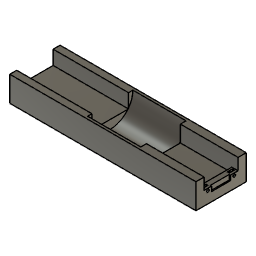
LabelStamp (Autodesk Fusion 360 design; units mm, degrees)
Autodesk Fusion 360 part; units mm, degrees
sketch "スケッチ1" plane through (0, 0, 0) normal (0, 0, 1) x (1, 0, 0)
  line L0 (0, 0) -> (148.1, 0)
  line L1 (148.1, 0) -> (148.1, 40)
  line L2 (148.1, 40) -> (0, 40)
  line L3 (0, 40) -> (0, 0)
  dimension "d1" = 148.1
  dimension "d2" = 40
  constraint horizontal L0
  constraint vertical L1
  constraint horizontal L2
  constraint vertical L3
  constraint coincident L0.start L3.end
  measures "d1" distance of L0.start L0.end
  measures "d2" distance of L0.start L2.end
extrude "押し出し1" add sketch "スケッチ1" along normal blind 8.8
sketch "スケッチ2" plane through (0, 0, 8.8) normal (0, 0, 1) x (-1, 0, 0)
  line L0 (0, -40) -> (0, 0)
  line L1 (0, 0) -> (-148.1, 0)
  line L2 (-148.1, 0) -> (-148.1, -40)
  line L3 (-148.1, -40) -> (0, -40)
  line L4 (-148.1, -40) -> (-102.2, -40)
  line L5 (-102.2, -40) -> (-102.2, -33.5)
  line L6 (-102.2, -33.5) -> (-148.1, -33.5)
  line L7 (-148.1, -33.5) -> (-148.1, -40)
  line L8 (-148.1, 0) -> (-102.2, 0)
  line L9 (-102.2, 0) -> (-102.2, -6.5)
  line L10 (-102.2, -6.5) -> (-148.1, -6.5)
  line L11 (-148.1, -6.5) -> (-148.1, 0)
  line L12 (0, -40) -> (-59.9, -40)
  line L13 (-59.9, -40) -> (-59.9, -34.5)
  line L14 (-59.9, -34.5) -> (0, -34.5)
  line L15 (0, -34.5) -> (0, -40)
  line L16 (0, 0) -> (-59.9, 0)
  line L17 (-59.9, 0) -> (-59.9, -5.5)
  line L18 (-59.9, -5.5) -> (0, -5.5)
  line L19 (0, -5.5) -> (0, 0)
  line L20 (-59.9, -40) -> (-102.2, -40)
  line L21 (-102.2, -40) -> (-102.2, 0)
  line L22 (-102.2, 0) -> (-59.9, 0)
  line L23 (-59.9, 0) -> (-59.9, -40)
  dimension "d5" = 45.9
  dimension "d6" = 6.5
  dimension "d7" = 45.9
  dimension "d8" = 6.5
  dimension "d9" = 59.9
  dimension "d10" = 5.5
  dimension "d11" = 59.9
  dimension "d12" = 5.5
  constraint horizontal L4
  constraint vertical L5
  constraint horizontal L6
  constraint vertical L7
  constraint coincident L2.end L3.start
  constraint horizontal L8
  constraint vertical L9
  constraint horizontal L10
  constraint vertical L11
  constraint coincident L1.end L2.start
  constraint horizontal L12
  constraint vertical L13
  constraint horizontal L14
  constraint vertical L15
  constraint coincident L0.start L3.end
  constraint horizontal L16
  constraint vertical L17
  constraint horizontal L18
  constraint vertical L19
  constraint coincident L0.end L1.start
  constraint horizontal L20
  constraint vertical L21
  constraint horizontal L22
  constraint vertical L23
  measures "d5" distance of L2.end L4.end
  measures "d6" distance of L2.end L6.end
  measures "d7" distance of L1.end L8.end
  measures "d8" distance of L1.end L10.end
  measures "d9" distance of L0.start L12.end
  measures "d10" distance of L0.start L14.end
  measures "d11" distance of L0.end L16.end
  measures "d12" distance of L0.end L18.end
extrude "押し出し2" add sketch "スケッチ2" along normal blind 11.2 contours L0 L3 L12 L13 L14 L15 L23 | L1 L3 L5 L9 L13 L17 L20 L21 L22 L23 | L0 L1 L16 L17 L18 L19 L23 | L2 L3 L4 L5 L6 L7 L21 | L1 L2 L8 L9 L10 L11 L21
extrude "押し出し5" cut 1 faces at (117.5, 24.5, 8.8) along direction (0, 0, -1) blind 1.8
sketch "スケッチ4" plane through (0, 0, 7) normal (0, 0, 1) x (-1, 0, 0)
  line L0 (-102.2, -6.5) -> (-148.1, -6.5)
  line L1 (-148.1, -6.5) -> (-148.1, -33.5)
  line L2 (-148.1, -33.5) -> (-102.2, -33.5)
  line L3 (-102.2, -33.5) -> (-102.2, -6.5)
  line L4 (-148.1, -33.5) -> (-143.1, -33.5)
  line L5 (-143.1, -33.5) -> (-143.1, -6.5)
  line L6 (-143.1, -6.5) -> (-148.1, -6.5)
  line L7 (-148.1, -6.5) -> (-148.1, -33.5)
  dimension "d22" = 5
  constraint horizontal L4
  constraint vertical L5
  constraint horizontal L6
  constraint vertical L7
  constraint coincident L1.end L2.start
  measures "d22" distance of L1.end L4.end
extrude "押し出し6" add sketch "スケッチ4" along normal blind 3.8 contours L0 L1 L2 L4 L5 L6 L7
sketch "スケッチ7" plane through (102.2, 0, 0) normal (1, 0, 0) x (0, 1, 0)
  line L0 (33.5, 7) -> (33.5, 20)
  line L1 (33.5, 20) -> (6.5, 20)
  line L2 (6.5, 20) -> (6.5, 7)
  line L3 (6.5, 7) -> (33.5, 7)
  circle A0 centre (20, 20) radius 18
  dimension "d28" = 36
  constraint midpoint L1 A0.centre
  measures "d28" diameter of A0
extrude "押し出し8" cut sketch "スケッチ7" against normal blind 42.3 contours L0 L1 L2 L3 A0 | L0 L1 L2 A0 | L3 A0
sketch "スケッチ8" plane through (0, 0, 10.8) normal (0, 0, 1) x (-1, 0, 0)
  line L0 (-148.1, -6.5) -> (-148.1, -33.5)
  line L1 (-148.1, -33.5) -> (-143.1, -33.5)
  line L2 (-143.1, -33.5) -> (-143.1, -6.5)
  line L3 (-143.1, -6.5) -> (-148.1, -6.5)
  line L4 (-144.5, -32.5) -> (-146.1, -32.5)
  line L5 (-146.1, -32.5) -> (-146.1, -28.5)
  line L6 (-146.1, -28.5) -> (-144.5, -28.5)
  line L7 (-144.5, -28.5) -> (-144.5, -32.5)
  line L8 (-146.1, -7.5) -> (-144.5, -7.5)
  line L9 (-144.5, -7.5) -> (-144.5, -11.5)
  line L10 (-144.5, -11.5) -> (-146.1, -11.5)
  line L11 (-146.1, -11.5) -> (-146.1, -7.5)
  dimension "d31" = 1.6
  dimension "d32" = 4
  dimension "d33" = 1.4
  dimension "d34" = 1
  dimension "d35" = 1.6
  dimension "d36" = 4
  dimension "d37" = 1
  dimension "d38" = 1.4
  constraint horizontal L4
  constraint vertical L5
  constraint horizontal L6
  constraint vertical L7
  constraint horizontal L8
  constraint vertical L9
  constraint horizontal L10
  constraint vertical L11
  measures "d31" distance of L4.start L4.end
  measures "d32" distance of L4.start L6.end
  measures "d33" distance of L2 L7
  measures "d34" distance of L1 L4
  measures "d35" distance of L8.start L8.end
  measures "d36" distance of L8.start L10.end
  measures "d37" distance of L3 L8
  measures "d38" distance of L2 L9
extrude "押し出し9" cut sketch "スケッチ8" against normal blind 4 contours L4 L5 L6 L7 | L8 L9 L10 L11
sketch "スケッチ9" plane through (148.1, 0, 0) normal (1, 0, 0) x (0, 1, 0)
  line L0 (33.5, 20) -> (33.5, 10.8)
  line L1 (33.5, 10.8) -> (6.5, 10.8)
  line L2 (6.5, 10.8) -> (6.5, 20)
  line L3 (6.5, 20) -> (0, 20)
  line L4 (0, 20) -> (0, 0)
  line L5 (0, 0) -> (40, 0)
  line L6 (40, 0) -> (40, 20)
  line L7 (40, 20) -> (33.5, 20)
  circle A0 centre (9.5, 9) radius 1.05
  circle A1 centre (30.5, 9) radius 1.05
  point P0 (30.5, 9)
  point P1 (9.5, 9)
  dimension "d41" = 9.5
  dimension "d42" = 1.8
  dimension "d43" = 9.5
  dimension "d44" = 1.8
  dimension "d45" = 2.1
  dimension "d46" = 2.1
  constraint coincident P1 A0.centre
  constraint coincident P0 A1.centre
  measures "d41" distance of L6 P0
  measures "d42" distance of L1 P0
  measures "d43" distance of L4 P1
  measures "d44" distance of L1 P1
  measures "d45" diameter of A0
  measures "d46" diameter of A1
extrude "押し出し10" cut sketch "スケッチ9" against normal blind 5 contours A0 | A1
sketch "スケッチ10" plane through (148.1, 0, 0) normal (1, 0, 0) x (0, 1, 0)
  circle A0 centre (9.5, 9) radius 1.05
  circle A1 centre (30.5, 9) radius 1.05
  line L0 (33.5, 20) -> (33.5, 10.8)
  line L1 (33.5, 10.8) -> (6.5, 10.8)
  line L2 (6.5, 10.8) -> (6.5, 20)
  line L3 (6.5, 20) -> (0, 20)
  line L4 (0, 20) -> (0, 0)
  line L5 (0, 0) -> (40, 0)
  line L6 (40, 0) -> (40, 20)
  line L7 (40, 20) -> (33.5, 20)
  line L8 (12.5, 10.8) -> (27.5, 10.8)
  line L9 (27.5, 10.8) -> (27.5, 7)
  line L10 (27.5, 7) -> (12.5, 7)
  line L11 (12.5, 7) -> (12.5, 10.8)
  dimension "d49" = 15
  dimension "d50" = 3.8
  dimension "d51" = 12.5
  constraint horizontal L8
  constraint vertical L9
  constraint horizontal L10
  constraint vertical L11
  constraint coincident L1 L8.start
  measures "d49" distance of L8.start L8.end
  measures "d50" distance of L8.start L10.end
  measures "d51" distance of L6 L9
extrude "押し出し11" cut sketch "スケッチ10" against normal blind 1 contours L1 L8 L9 L10 L11
